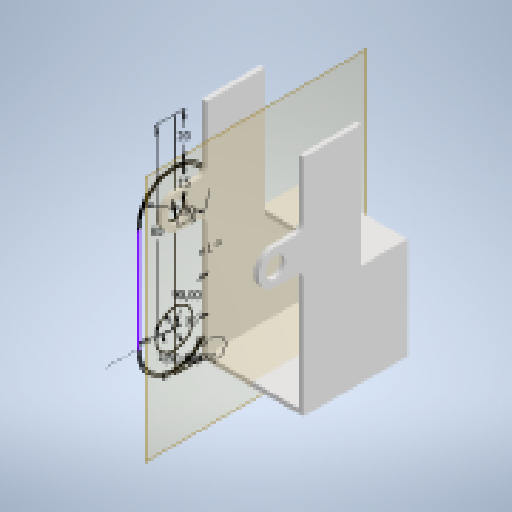
# Autodesk Inventor part: Tolva1
Saved by Autodesk Inventor 2023 (Build 270158000, 158)
## iProperties
Created: 2023-04-20
Part Number: Tolva1
Material: Genérico
Document SubType Name: Modeling
Designer: sergi
Density: 1 g/cm^3
Appearance: Valor por defecto
Author: sergi
Autodesk Inventor part; units mm, degrees
ref_plane "YZ Plane" through (0, 0, 0) normal (1, 0, 0) x (0, 1, 0)
ref_plane "XZ Plane" through (0, 0, 0) normal (0, 1, 0) x (-1, 0, 0)
sketch "Boceto1" plane through (0, 0, 0) normal (0, 0, 1) x (1, 0, 0)
  line L0 (0, 0) -> (40, 0)
  line L1 (40, 0) -> (40, -40)
  line L2 (40, -40) -> (0, -40)
  line L3 (0, -40) -> (0, 0)
  line L4 (-2, 2) -> (42, 2)
  line L5 (42, 2) -> (42, -42)
  line L6 (42, -42) -> (-2, -42)
  line L7 (-2, -42) -> (-2, 2)
  dimension "d0" = 40
  dimension "d1" = 40
  dimension "d2" = 2
  constraints: 16 end point, 4 parallel, 2 perpendicular, 1 horizontal, 3 other
  measures "d0" distance of L1.end L2.end
  measures "d1" distance of L0.end L1.end
  measures "d2" distance between parallel lines of L3 L7
extrude "Extrusión1" add sketch "Boceto1" along normal blind 40
sketch "Boceto3" plane through (-2, -42, 0) normal (-1, 0, 0) x (0, 0, 1)
  line L0 (40, 2) -> (40, 42) projected
  line L1 (0, 0) -> (40, 0) projected
  line L2 (40, 0) -> (57, 0)
  line L3 (40, 0) -> (57, 0) construction
  line L4 (57, 0) -> (57, 17)
  line L5 (57, 17) -> (57, 97)
  arc A0 (42, 17) -> (72, 17) centre (57, 17) ccw
  line L6 (57, 97) -> (57, 77)
  line L7 (57, 77) -> (57, 62)
  arc A1 (72, 62) -> (42, 62) centre (57, 62) ccw
  line L8 (42, 17) -> (42, 62)
  line L9 (42, 17) -> (87, 17) construction
  line L10 (72, 17) -> (72, 62)
  line L11 (41, 62) -> (41, 17)
  arc A2 (41, 17) -> (73, 17) centre (57, 17) ccw
  line L12 (73, 17) -> (73, 62)
  arc A3 (73, 62) -> (41, 62) centre (57, 62) ccw
  circle A4 centre (57, 17) radius 8
  circle A5 centre (57, 62) radius 4
  point P0 (0, 42)
  dimension "d20" = 17
  dimension "d21" = 0
  dimension "d22" = 17
  dimension "d23" = 90
  dimension "d24" = 80
  dimension "d25" = 30
  dimension "d26" = 20
  dimension "d27" = 15
  dimension "d28" = 30
  dimension "d29" = 90
  dimension "d30" = 1
  dimension "d31" = 16
  dimension "d32" = 8
  constraints: 22 end point, 8 point on circle, 6 centre point, 4 coincident, 3 horizontal, 3 point on line, 2 equal length, 1 perpendicular, 1 tangent, 3 other
  measures "d20" distance of L1.end L2.end
  measures "d21" distance between parallel lines of L2 L3
  measures "d22" distance of L2.end L4.end
  measures "d23" angle of L4 L2
  measures "d24" distance of L4.end L5.end
  measures "d25" diameter of A0
  measures "d26" distance of L5.end L6.end
  measures "d27" distance of L6.end L7.end
  measures "d28" diameter of A1
  measures "d29" angle of L9 L8
  measures "d30" distance between parallel lines of L8 L11
  measures "d31" diameter of A4
  measures "d32" diameter of A5
sketch "Boceto4" plane through (0, 0, 40) normal (0, 0, 1) x (1, 0, 0)
  line L0 (0, 0) -> (40, 0)
  line L1 (40, 0) -> (40, 1.9053)
  line L2 (0, 1.9053) -> (0, 0)
  line L3 (42, 2) -> (-2, 2) projected
  line L4 (0, 0) -> (40, 0)
  line L5 (40, 0) -> (40, 2)
  line L6 (40, 2) -> (0, 2)
  line L7 (0, 2) -> (0, 0)
  dimension "d35" = 40
  constraints: 14 end point, 3 parallel, 2 horizontal, 2 perpendicular, 1 point on line
  measures "d35" distance of L6.end L5.end
extrude "Extrusión2" cut sketch "Boceto4" against normal blind 20
sketch "Boceto5" plane through (-2, 2, 0) normal (0, 1, 0) x (1, 0, 0)
  line L0 (2, -40) -> (0, -40) projected
  line L1 (2, -20) -> (42, -20) projected
  line L2 (0, -40) -> (2, -40)
  line L3 (2, -40) -> (2, -20)
  line L4 (2, -20) -> (0, -20)
  line L5 (0, -20) -> (0, -40)
  line L6 (44, 0) -> (44, -40) projected
  line L7 (42, -20) -> (44, -20)
  line L8 (44, -20) -> (44, -40)
  line L9 (44, -40) -> (42, -40)
  line L10 (42, -40) -> (42, -20)
  point P0 (2, 0)
  constraints: 16 end point, 4 parallel, 2 horizontal, 2 perpendicular
extrude "Extrusión3" add sketch "Boceto5" along normal blind 53
sketch "Boceto6" plane through (0, 0, 40) normal (0, 0, 1) x (1, 0, 0)
  line L0 (0, -40) -> (0, 55) projected
  line L1 (-2, 55) -> (0, 55) projected
  line L2 (-2, -42) -> (-2, 55) projected
  line L3 (-2, -42) -> (42, -42) projected
  line L4 (42, -42) -> (42, 55) projected
  line L5 (40, 55) -> (42, 55) projected
  line L6 (40, -40) -> (40, 55) projected
  line L7 (40, -40) -> (0, -40) projected
  point P0 (0, 0)
extrude "Extrusión4" add sketch "Boceto6" along normal blind 5
sketch "Boceto7" plane through (-2, -42, 0) normal (-1, 0, 0) x (0, 0, 1)
  line L0 (61.25, 64.0484) -> (52.75, 59.9516) construction
  line L1 (52.75, 64.0484) -> (61.25, 59.9516) construction
  line L2 (0, 44) -> (0, 0) projected
  line L3 (0, 0) -> (45, 0) projected
  line L4 (45, 97) -> (45, 0) projected
  line L5 (20, 97) -> (45, 97) projected
  line L6 (20, 44) -> (20, 97) projected
  line L7 (0, 44) -> (20, 44) projected
  circle A0 centre (57, 62) radius 4.25
  circle A1 centre (57, 62) radius 7.5
  line L8 (45, 2) -> (45, 97) projected
  line L9 (57, 69.5) -> (45, 69.5)
  line L10 (57, 54.5) -> (45, 54.5)
  point P0 (0, 42)
  dimension "d40" = 8.5
  dimension "d49" = 15
  constraints: 8 end point, 2 centre point, 2 coincident, 2 midpoint, 2 point on circle, 2 point on line, 1 horizontal, 1 perpendicular, 1 other
  measures "d40" distance of L1.end L0.end
  measures "d49" diameter of A1
extrude "Extrusión5" add sketch "Boceto7" against normal blind 2 contours L4 L9 A1 L10 | A1
fillet "Empalme1" radius 3 2 edges at (-1, 12.5, 45) (-1, 27.5, 45)
ref_plane "Plano de trabajo1" through (20, -40, 0) normal (1, 0, 0) x (0, 0, -1)
mirror "Simetría1" about plane through (20, -40, 0) normal (1, 0, 0) of "Extrusión5", "Empalme1"
sketch "Boceto8" plane through (40, -40, 0) normal (-1, 0, 0) x (0, 0, 1)
  line L0 (20, 42) -> (20, 95) projected
  line L1 (20, 95) -> (45, 95)
  line L2 (45, 95) -> (45, 93)
  line L3 (45, 93) -> (20, 93)
  line L4 (20, 93) -> (20, 95)
  point P0 (0, 40)
  dimension "d53" = 2
  constraints: 8 end point, 2 parallel, 1 horizontal, 1 perpendicular
  measures "d53" distance of L1.end L2.end
extrude "Extrusión6" add sketch "Boceto8" along normal blind 40
sketch "Boceto9" plane through (-2, 2, 0) normal (0, 1, 0) x (1, 0, 0)
  line L0 (42, -20) -> (44, -20) projected
  line L1 (44, 0) -> (44, -20) projected
  line L2 (44, 0) -> (0, 0) projected
  line L3 (0, 0) -> (0, -20) projected
  line L4 (0, -20) -> (2, -20) projected
  line L5 (2, -20) -> (42, -20) projected
  line L6 (0, -20) -> (0, -15)
  line L7 (0, -15) -> (44, -15)
  line L8 (22, -15) -> (12, -15)
  line L9 (22, -15) -> (32, -15) construction
  line L10 (12, -15) -> (22, -15)
  circle A0 centre (12, -15) radius 1.5
  circle A1 centre (32, -15) radius 1.5
  point P0 (2, 0)
  dimension "d56" = 5
  dimension "d57" = 10
  dimension "d58" = 180
  dimension "d59" = 3
  dimension "d60" = 3
  constraints: 10 end point, 3 collinear, 2 centre point, 2 coincident, 2 point on line, 1 horizontal, 1 midpoint, 1 perpendicular
  measures "d56" distance of L3.end L6.end
  measures "d57" distance of L8.start L8.end
  measures "d58" angle of L8 L9
  measures "d59" diameter of A0
  measures "d60" diameter of A1
hole "Agujero1" at (10, 2, 15) at (30, 2, 15) direction (0, -1, 0) diameter 3 depth 2 tip angle 118
sketch "Boceto10" plane through (-2, 55, 0) normal (0, 1, 0) x (1, 0, 0)
  line L0 (0, -20) -> (0, -45) projected
  line L1 (44, -45) -> (0, -45) projected
  line L2 (44, -20) -> (44, -45) projected
  point P0 (2, 0)
  point P1 (10, -32.5)
  point P2 (34, -32.5)
  dimension "d68" = 10
  dimension "d69" = 12.5
  dimension "d70" = 10
  dimension "d71" = 12.5
  measures "d68" distance from line of L0 point (10, -32.5)
  measures "d69" distance from line of L1 point (10, -32.5)
  measures "d70" distance from line of L2 point (34, -32.5)
  measures "d71" distance from line of L1 point (34, -32.5)
hole "Agujero2" at (8, 55, 32.5) at (32, 55, 32.5) direction (0, -1, 0) diameter 3 end through all
sketch "Boceto11" plane through (-2, -42, 0) normal (-1, 0, 0) x (0, 0, 1)
  circle A0 centre (37, 21.25) radius 1.5 projected
  circle A1 centre (37, 12.75) radius 1.5 projected
  point P0 (0, 42)
hole "Agujero3" at (-2, -29.25, 37) at (-2, -20.75, 37) direction (1, 0, 0) diameter 3 end through all
fillet "Empalme2" radius 3 2 edges at (41, 2, 20) (-1, 2, 20)
